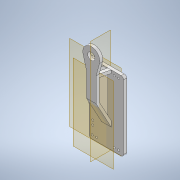
# Autodesk Inventor part: Fastener
Saved by Autodesk Inventor 2022 (Build 260153000, 153)
## iProperties
Created: 2023-10-19
Part Number: Fastener
Material: Типовые
Document SubType Name: Modeling
Designer: user
Density: 1 g/cm^3
Appearance: По умолчанию
Author: user
Autodesk Inventor part; units mm, degrees
ref_plane "YZ Plane" through (0, 0, 0) normal (1, 0, 0) x (0, 1, 0)
ref_plane "XZ Plane" through (0, 0, 0) normal (0, 1, 0) x (-1, 0, 0)
ref_plane "XY Plane" through (0, 0, 0) normal (0, 0, 1) x (1, 0, 0)
ref_plane "РабПлоскость1" through (0, 0, 0) normal (0, 0, 1) x (1, 0, 0)
sketch "Эскиз1" plane through (0, 0, 0) normal (0, 0, 1) x (1, 0, 0)
  line L0 (15.9535, 22.685) -> (15.9535, 17.285) projected
  line L1 (15.9535, 17.285) -> (5.5535, 17.285) projected
  line L2 (5.5535, 17.285) -> (5.5535, 22.685) projected
  line L3 (5.5535, 22.685) -> (15.9535, 22.685) projected
  line L4 (15.9535, -17.315) -> (15.9535, -22.715) projected
  line L5 (15.9535, -22.715) -> (5.5535, -22.715) projected
  line L6 (5.5535, -22.715) -> (5.5535, -17.315) projected
  line L7 (5.5535, -17.315) -> (15.9535, -17.315) projected
  arc A0 (-2.3465, 28.685) -> (-4.3465, 26.685) centre (-2.3465, 26.685) ccw projected
  line L8 (-4.3465, 12.1) -> (-4.3465, 26.685) projected
  arc A1 (-5.6809, 10.2141) -> (-4.3465, 12.1) centre (-6.3465, 12.1) ccw projected
  line L9 (-11.5122, 8.156) -> (-5.6809, 10.2141) projected
  arc A2 (-11.5122, 8.156) -> (-12.8465, 6.27) centre (-10.8465, 6.27) ccw projected
  line L10 (-12.8465, -1.915) -> (-12.8465, 6.27) projected
  arc A3 (-12.8465, -1.915) -> (-10.8465, -3.915) centre (-10.8465, -1.915) ccw projected
  line L11 (-4.6465, -3.915) -> (-10.8465, -3.915) projected
  arc A4 (-2.6465, -5.915) -> (-4.6465, -3.915) centre (-4.6465, -5.915) ccw projected
  line L12 (-2.6465, -26.715) -> (-2.6465, -5.915) projected
  arc A5 (-2.6465, -26.715) -> (-0.6465, -28.715) centre (-0.6465, -26.715) ccw projected
  line L13 (23.8535, -28.715) -> (-0.6465, -28.715) projected
  arc A6 (23.8535, -28.715) -> (25.8535, -26.715) centre (23.8535, -26.715) ccw projected
  line L14 (25.8535, 26.685) -> (25.8535, -26.715) projected
  arc A7 (25.8535, 26.685) -> (23.8535, 28.685) centre (23.8535, 26.685) ccw projected
  line L15 (-2.3465, 28.685) -> (23.8535, 28.685) projected
  circle A8 centre (18.0535, 25.685) radius 0.8 projected
  circle A9 centre (21.6535, 25.685) radius 0.8 projected
  circle A10 centre (21.6535, -25.715) radius 0.8 projected
  circle A11 centre (18.0535, -25.715) radius 0.8 projected
  circle A12 centre (0.3535, -18.515) radius 0.8 projected
  circle A13 centre (0.3535, -14.915) radius 0.8 projected
  circle A14 centre (-1.3465, 16.885) radius 0.8 projected
  circle A15 centre (-1.3465, 20.485) radius 0.8 projected
  circle A16 centre (-0.1465, 25.685) radius 0.8 projected
  circle A17 centre (3.4535, 25.685) radius 0.8 projected
  circle A18 centre (-0.1465, -25.715) radius 0.8 projected
  circle A19 centre (3.4535, -25.715) radius 0.8 projected
  line L16 (-4.3465, 12.1) -> (-2.6465, -5.915)
  circle A20 centre (51.6035, 35.685) radius 3
  circle A21 centre (51.6035, 35.685) radius 6
  line L17 (11.6035, -28.715) -> (11.6035, 28.685) construction
  line L18 (56.9244, 32.9123) -> (25.8535, -26.715)
  line L19 (50.1799, 41.5137) -> (-2.3465, 28.685)
  point P0 (0, 0)
  point P1 (-2.6818, -5.5409)
  dimension "d11" = 6
  dimension "d12" = 12
  dimension "d13" = 7
  dimension "d14" = 40
  constraints: 8 end point, 2 centre point, 2 point on circle, 2 tangent, 1 coincident, 1 midpoint, 1 perpendicular, 1 point on line
  measures "d11" diameter of A20
  measures "d12" diameter of A21
  measures "d13" distance from line of L15 A20.centre
  measures "d14" distance from line of A20.centre L17
extrude "Выдавливание1" add sketch "Эскиз1" along normal blind 2.5 contours L0 L1 L2 L3 | L4 L5 L6 L7 | L15 A7 L14 A6 L13 A5 L12 A4 L16 L8 A0
ref_plane "РабПлоскость4" through (0, 0, 12.5) normal (0, 0, 1) x (1, 0, 0)
sketch "Эскиз7" plane through (0, 0, 12.5) normal (0, 0, 1) x (1, 0, 0)
  circle A0 centre (11.6035, 42.685) radius 3
  circle A1 centre (11.6035, 42.685) radius 7
  line L0 (18.3597, 40.8537) -> (15.6035, 30.685)
  line L1 (15.6035, 30.685) -> (15.6035, 10.685)
  line L2 (15.6035, 10.685) -> (7.6035, 10.685)
  line L3 (7.6035, 10.685) -> (7.6035, 30.685)
  line L4 (7.6035, 30.685) -> (4.8473, 40.8537)
  line L5 (-0.6465, -28.715) -> (23.8535, -28.715) projected
  line L6 (11.6035, -28.715) -> (11.6035, 28.685) construction
  line L7 (23.8535, 28.685) -> (-2.3465, 28.685) projected
  point P0 (0, 0)
  point P1 (11.6035, 10.685)
  dimension "d46" = 6
  dimension "d47" = 14
  dimension "d48" = 32
  dimension "d49" = 4
  dimension "d50" = 18
  dimension "d51" = 20
  dimension "d52" = 20
  constraints: 12 end point, 3 point on line, 2 centre point, 2 midpoint, 2 perpendicular, 2 point on circle, 2 tangent, 2 vertical, 1 coincident
  measures "d46" diameter of A0
  measures "d47" diameter of A1
  measures "d48" distance from line of A0.centre L2
  measures "d49" distance between parallel lines of L6 L1
  measures "d50" distance between parallel lines of L7 L2
  measures "d51" distance from line of L0.end L2
  measures "d52" distance from line of L3.end L2
extrude "Выдавливание5" add sketch "Эскиз7" along normal blind 2.5
ref_plane "РабПлоскость5" through (11.6035, 10.685, 12.5) normal (1, 0, 0) x (0, 0, -1)
sketch "Эскиз8" plane through (11.6035, 10.685, 12.5) normal (1, 0, 0) x (0, 0, -1)
  line L0 (0, 20) -> (0, 30.1687) projected
  line L1 (10, 18) -> (10, 16) projected
  line L2 (0, 20) -> (10, 18)
  line L3 (-2.5, 20) -> (-2.5, 0) projected
  line L4 (-2.5, 0) -> (10, -23)
  line L5 (10, -37.4) -> (10, 16) projected
  line L6 (0, 0) -> (0, 20) projected
  line L7 (0, 0) -> (-2.5, 0) projected
  line L8 (0, 20) -> (0, 0) projected
  line L9 (0, 0) -> (10, -18.4)
  line L10 (10, -16.6) -> (10, -37.4) projected
  line L11 (0, 17.4505) -> (10, 15.4505)
  line L12 (10, 16) -> (10, 1.415) projected
  line L13 (12.5, 18) -> (10, 18) projected
  line L14 (10, 18) -> (0, 25.5)
  point P0 (12.5, -10.685)
  dimension "d55" = 23
  dimension "d56" = 2.5
  dimension "d61" = 5.5
  constraints: 10 end point, 6 point on line, 2 parallel
  measures "d55" vertical distance of L3.end L4.end
  measures "d56" distance between parallel lines of L2 L11
  measures "d61" distance of L0.start L14.end
extrude "Выдавливание6" add sketch "Эскиз8" along normal mid plane 2.5 contours L0 L14 L2 | L11 L5 L9 L6
extrude "Выдавливание7" add sketch "Эскиз8" along normal mid plane 8 contours L2 L1 L5 L11 L6 | L9 L5 L4 L7
